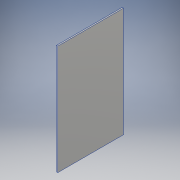
# Autodesk Inventor part: CAR_031_VersaplanetaryMountPlate
Saved by Autodesk Inventor 2018 (Build 220112000, 112)
## iProperties
Created: 2020-02-06
Part Number: CAR_031_VersaplanetaryMountPlate
Material: Aluminum 6061
Document SubType Name: Modeling
Designer: user
Mass: 41.4798 g
Surface Area: 200 cm^2
Volume: 15.3629 cm^3
Density: 2.7 g/cm^3
Appearance: Aluminum - Flat
Author: user
Autodesk Inventor part; units mm, degrees
ref_plane "YZ Plane" through (0, 0, 0) normal (1, 0, 0) x (0, 1, 0)
ref_plane "XZ Plane" through (0, 0, 0) normal (0, 1, 0) x (-1, 0, 0)
ref_plane "XY Plane" through (0, 0, 0) normal (0, 0, 1) x (1, 0, 0)
sketch "Sketch1" plane through (0, 0, 0) normal (1, 0, 0) x (0, 1, 0)
  line L0 (0, 0) -> (127, 0)
  line L1 (127, 0) -> (127, -76.2)
  line L2 (127, -76.2) -> (0, -76.2)
  line L3 (0, -76.2) -> (0, 0)
  dimension "d0" = 127
  dimension "d1" = 76.2
  constraints: 8 end point, 2 parallel, 1 horizontal, 1 perpendicular
  measures "d0" distance of L1.end L2.end
  measures "d1" distance of L0.end L1.end
extrude "Extrusion1" add sketch "Sketch1" along normal blind 1.5875
body "Solid1"
